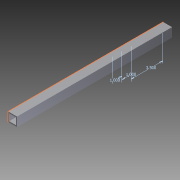
# Autodesk Inventor part: tower horizontal brace 17.5in
Saved by Autodesk Inventor 2011 SP1 (Build 150282100, 282)
## iProperties
Created: 2012-01-18
Part Number: tower horizontal brace 17.5in
Document SubType Name: Modeling
Designer: Christopher
Density: 1 g/cm^3
Author: Christopher
Autodesk Inventor part; units mm, degrees
ref_plane "YZ Plane" through (0, 0, 0) normal (1, 0, 0) x (0, 1, 0)
ref_plane "XZ Plane" through (0, 0, 0) normal (0, 1, 0) x (-1, 0, 0)
ref_plane "XY Plane" through (0, 0, 0) normal (0, 0, 1) x (1, 0, 0)
sketch "Sketch1" plane through (0, 0, 0) normal (0, 0, 1) x (1, 0, 0)
  line L0 (0, 0) -> (25.4, 0)
  line L1 (25.4, 0) -> (25.4, 25.4)
  line L2 (25.4, 25.4) -> (0, 25.4)
  line L3 (0, 25.4) -> (0, 0)
  line L4 (3.175, 3.175) -> (22.225, 3.175)
  line L5 (22.225, 3.175) -> (22.225, 22.225)
  line L6 (22.225, 22.225) -> (3.175, 22.225)
  line L7 (3.175, 22.225) -> (3.175, 3.175)
  dimension "d0" = 25.4
  dimension "d1" = 25.4
  dimension "d2" = 3.175
  constraints: 16 end point, 4 parallel, 2 perpendicular, 1 horizontal, 3 other
  measures "d0" distance of L1.end L2.end
  measures "d1" distance of L0.end L1.end
  measures "d2" distance between parallel lines of L3 L7
extrude "Extrusion1" add sketch "Sketch1" against normal blind 431.8
sketch "Sketch2" plane through (0, 0, 0) normal (-1, 0, 0) x (0, 0, 1)
  line L0 (-431.8, 25.4) -> (-431.8, 0) projected
  line L1 (0, 25.4) -> (0, 0) projected
  point P0 (-304.8, 12.7)
  point P1 (-279.4, 12.7)
  point P2 (-330.2, 12.7)
  point P3 (-101.6, 12.7)
  point P4 (-127, 12.7)
  point P5 (-152.4, 12.7)
  dimension "d5" = 25.4
  dimension "d6" = 25.4
  dimension "d7" = 101.6
  dimension "d25" = 101.6
  dimension "d26" = 25.4
  dimension "d27" = 25.4
  measures "d5" distance of point (-330.2, 12.7) point (-304.8, 12.7)
  measures "d6" distance of point (-279.4, 12.7) point (-304.8, 12.7)
  measures "d7" distance from line of L0 point (-330.2, 12.7)
  measures "d25" distance from line of L1 point (-101.6, 12.7)
  measures "d26" distance of point (-101.6, 12.7) point (-127, 12.7)
  measures "d27" distance of point (-152.4, 12.7) point (-127, 12.7)
hole "Hole1" at (0, 12.7, -304.8) at (0, 12.7, -279.4) at (0, 12.7, -330.2) at (0, 12.7, -127) at (0, 12.7, -101.6) at (0, 12.7, -152.4) direction (1, 0, 0) diameter 6.35 depth 25.4 tip angle 118
sketch "Sketch3" plane through (0, 0, 0) normal (0, -1, 0) x (1, 0, 0)
  line L0 (0, -431.8) -> (25.4, -431.8) projected
  line L1 (0, 0) -> (25.4, 0) projected
  point P0 (12.7, -330.2)
  point P1 (12.7, -355.6)
  point P2 (12.7, -381)
  point P3 (12.7, -50.8)
  point P4 (12.7, -76.2)
  point P5 (12.7, -101.6)
  point P6 (12.7, -419.1)
  point P7 (12.7, -12.7)
  dimension "d15" = 25.4
  dimension "d16" = 25.4
  dimension "d17" = 50.8
  dimension "d28" = 50.8
  dimension "d29" = 25.4
  dimension "d30" = 25.4
  dimension "d31" = 12.7
  dimension "d32" = 12.7
  measures "d15" distance of point (12.7, -355.6) point (12.7, -381)
  measures "d16" distance of point (12.7, -355.6) point (12.7, -330.2)
  measures "d17" distance from line of L0 point (12.7, -381)
  measures "d28" distance from line of L1 point (12.7, -50.8)
  measures "d29" distance of point (12.7, -50.8) point (12.7, -76.2)
  measures "d30" distance of point (12.7, -76.2) point (12.7, -101.6)
  measures "d31" distance from line of L0 point (12.7, -419.1)
  measures "d32" distance from line of L1 point (12.7, -12.7)
hole "Hole2" at (12.7, 0, -330.2) at (12.7, 0, -355.6) at (12.7, 0, -381) at (12.7, 0, -101.6) at (12.7, 0, -76.2) at (12.7, 0, -50.8) at (12.7, 0, -419.1) at (12.7, 0, -12.7) direction (0, 1, 0) diameter 6.35 depth 25.4 tip angle 118
body "Solid1"
